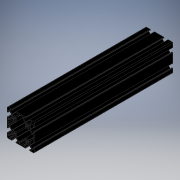
# Autodesk Inventor part: 20-4040-Black-203.2-CL
Saved by Autodesk Inventor 2019 (Build 230136000, 136)
## iProperties
Created: 2022-06-30
Part Number: 20-4040-Black-203.2-CL
Material: Generic
Catalog Web Link: www.cadenas.de
Description: 20-4040, 20-4040-Black-T-Slotted Profile - 20 Series
Vendor: 8020
Document SubType Name: Modeling
Designer: psAdmin
Manufacturer: 8020
Mass: 85.9678 g
Surface Area: 1092.07 cm^2
Volume: 85.9678 cm^3
Density: 1 g/cm^3
Appearance: PSOLRGB-0-0-0
Category: PARTsolutions
Company: 8020
Title: 20-4040-Black-203.2
Author: Cadenas PARTsolutions
Comments: T-Slotted Profile - 20 Series
PSOL_IDENT_0: {$CADENAS_DATA/23d-libs/8020/metric/profiles/20_series/20_4040.prj},206 {VTYP=3D},{NB=20-4040-Black-
PSOL_IDENT_1: 203.2-CL},{LINA=20-4040-Black-203.2},{NN=20-4040, 20-4040-Black},{DATE=31.07.2020 09:21:32},{GEOMDAT
PSOL_IDENT_2: E=09.02.2018 15:36:41},{VERSION=},{LINEID=10},{WBVAR=FIN,LS,L},{WBNUMERIC=L}  {NB=20-4040-Black-203.
PSOL_IDENT_3: 2-CL},{LINA=20-4040-Black-203.2},{KT=DUMMY},{PN=20-4040-Black-203.2},{PN1=20-4040},{FIN=BA},{LS=-CL}
PSOL_IDENT_4: ,{L=203.20},{SERIES=20-4040},{MAT=6105-T5 Aluminum},{W=1.1727},{LALG=[25:6000/0.05]},{MIX=7.8220},{M
PSOL_IDENT_5: IY=7.8220},{EA=4.2221},{COLOR=0,0,0}
NB: 20-4040-Black-203.2-CL
NN: 20-4040, 20-4040-Black
NT: T-Slotted Profile - 20 Series
NBSYN: $PN.$LS.
LINA: 20-4040-Black-203.2
CATALOG: 80/20
PN: 20-4040-Black-203.2
FIN: Black Anodize
LS: Custom Length
L: 203.2
SERIES: 20-4040
MAT: 6105-T5 Aluminum
W: 1.1727
MIX: 7.8220
MIY: 7.8220
EA: 4.2221
SUPPLIER: 8020
ARTICLENO: 20-4040-Black-203.2-CL
BOMINFO: 20-4040-Black-203.2
CREATOR: CADENAS GmbH
Autodesk Inventor part; units mm, degrees
ref_plane "YZ Plane" through (0, 0, 0) normal (1, 0, 0) x (0, 1, 0)
ref_plane "XZ Plane" through (0, 0, 0) normal (0, 1, 0) x (-1, 0, 0)
ref_plane "XY Plane" through (0, 0, 0) normal (0, 0, 1) x (1, 0, 0)
sketch "Sketch_1" plane through (0, 0, 0) normal (0, 0, 1) x (1, 0, 0)
  line L0 (-20, 28.5) -> (-20, 23.138)
  arc A0 (-20, 23.138) -> (-19.492, 22.63) centre (-19.492, 23.138) ccw
  line L1 (-19.492, 22.63) -> (-19.008, 22.63)
  arc A1 (-19.008, 22.63) -> (-18.5, 23.138) centre (-19.008, 23.138) ccw
  line L2 (-18.5, 23.138) -> (-18.5, 25.487)
  arc A2 (-17.992, 25.995) -> (-18.5, 25.487) centre (-17.992, 25.487) ccw
  line L3 (-17.992, 25.995) -> (-17.2659, 25.995)
  arc A3 (-16.9067, 25.8462) -> (-17.2659, 25.995) centre (-17.2659, 25.487) ccw
  line L4 (-16.9067, 25.8462) -> (-13.8038, 22.7433)
  arc A4 (-13.655, 22.3841) -> (-13.8038, 22.7433) centre (-14.163, 22.3841) ccw
  line L5 (-13.655, 22.3841) -> (-13.655, 17.6162)
  arc A5 (-13.8038, 17.257) -> (-13.655, 17.6162) centre (-14.163, 17.6162) ccw
  line L6 (-13.8038, 17.257) -> (-16.907, 14.1538)
  arc A6 (-17.2662, 14.005) -> (-16.907, 14.1538) centre (-17.2662, 14.513) ccw
  line L7 (-17.2662, 14.005) -> (-17.992, 14.005)
  arc A7 (-18.5, 14.513) -> (-17.992, 14.005) centre (-17.992, 14.513) ccw
  line L8 (-18.5, 14.513) -> (-18.5, 16.862)
  arc A8 (-18.5, 16.862) -> (-19.008, 17.37) centre (-19.008, 16.862) ccw
  line L9 (-19.008, 17.37) -> (-19.492, 17.37)
  arc A9 (-19.492, 17.37) -> (-20, 16.862) centre (-19.492, 16.862) ccw
  line L10 (-20, 16.862) -> (-20, 3.138)
  arc A10 (-20, 3.138) -> (-19.492, 2.63) centre (-19.492, 3.138) ccw
  line L11 (-19.492, 2.63) -> (-19.008, 2.63)
  arc A11 (-19.008, 2.63) -> (-18.5, 3.138) centre (-19.008, 3.138) ccw
  line L12 (-18.5, 3.138) -> (-18.5, 5.487)
  arc A12 (-17.992, 5.995) -> (-18.5, 5.487) centre (-17.992, 5.487) ccw
  line L13 (-17.992, 5.995) -> (-17.2662, 5.995)
  arc A13 (-16.907, 5.8462) -> (-17.2662, 5.995) centre (-17.2662, 5.487) ccw
  line L14 (-16.907, 5.8462) -> (-13.8038, 2.743)
  arc A14 (-13.655, 2.3838) -> (-13.8038, 2.743) centre (-14.163, 2.3838) ccw
  line L15 (-13.655, 2.3838) -> (-13.655, -2.3841)
  arc A15 (-13.8038, -2.7433) -> (-13.655, -2.3841) centre (-14.163, -2.3841) ccw
  line L16 (-13.8038, -2.7433) -> (-16.9067, -5.8462)
  arc A16 (-17.2659, -5.995) -> (-16.9067, -5.8462) centre (-17.2659, -5.487) ccw
  line L17 (-17.2659, -5.995) -> (-17.992, -5.995)
  arc A17 (-18.5, -5.487) -> (-17.992, -5.995) centre (-17.992, -5.487) ccw
  line L18 (-18.5, -5.487) -> (-18.5, -3.138)
  arc A18 (-18.5, -3.138) -> (-19.008, -2.63) centre (-19.008, -3.138) ccw
  line L19 (-19.008, -2.63) -> (-19.492, -2.63)
  arc A19 (-19.492, -2.63) -> (-20, -3.138) centre (-19.492, -3.138) ccw
  line L20 (-20, -3.138) -> (-20, -8.5)
  arc A20 (-20, -8.5) -> (-18.5, -10) centre (-18.5, -8.5) ccw
  line L21 (-18.5, -10) -> (-13.138, -10)
  arc A21 (-13.138, -10) -> (-12.63, -9.492) centre (-13.138, -9.492) ccw
  line L22 (-12.63, -9.492) -> (-12.63, -9.008)
  arc A22 (-12.63, -9.008) -> (-13.138, -8.5) centre (-13.138, -9.008) ccw
  line L23 (-13.138, -8.5) -> (-15.487, -8.5)
  arc A23 (-15.995, -7.992) -> (-15.487, -8.5) centre (-15.487, -7.992) ccw
  line L24 (-15.995, -7.992) -> (-15.995, -7.2662)
  arc A24 (-15.8462, -6.907) -> (-15.995, -7.2662) centre (-15.487, -7.2662) ccw
  line L25 (-15.8462, -6.907) -> (-12.743, -3.8038)
  arc A25 (-12.3838, -3.655) -> (-12.743, -3.8038) centre (-12.3838, -4.163) ccw
  line L26 (-12.3838, -3.655) -> (-7.6159, -3.655)
  arc A26 (-7.2567, -3.8038) -> (-7.6159, -3.655) centre (-7.6159, -4.163) ccw
  line L27 (-7.2567, -3.8038) -> (-4.1538, -6.9067)
  arc A27 (-4.005, -7.2659) -> (-4.1538, -6.9067) centre (-4.513, -7.2659) ccw
  line L28 (-4.005, -7.2659) -> (-4.005, -7.992)
  arc A28 (-4.513, -8.5) -> (-4.005, -7.992) centre (-4.513, -7.992) ccw
  line L29 (-4.513, -8.5) -> (-6.862, -8.5)
  arc A29 (-6.862, -8.5) -> (-7.37, -9.008) centre (-6.862, -9.008) ccw
  line L30 (-7.37, -9.008) -> (-7.37, -9.492)
  arc A30 (-7.37, -9.492) -> (-6.862, -10) centre (-6.862, -9.492) ccw
  line L31 (-6.862, -10) -> (6.862, -10)
  arc A31 (6.862, -10) -> (7.37, -9.492) centre (6.862, -9.492) ccw
  line L32 (7.37, -9.492) -> (7.37, -9.008)
  arc A32 (7.37, -9.008) -> (6.862, -8.5) centre (6.862, -9.008) ccw
  line L33 (6.862, -8.5) -> (4.513, -8.5)
  arc A33 (4.005, -7.992) -> (4.513, -8.5) centre (4.513, -7.992) ccw
  line L34 (4.005, -7.992) -> (4.005, -7.2659)
  arc A34 (4.1538, -6.9067) -> (4.005, -7.2659) centre (4.513, -7.2659) ccw
  line L35 (4.1538, -6.9067) -> (7.2567, -3.8038)
  arc A35 (7.6159, -3.655) -> (7.2567, -3.8038) centre (7.6159, -4.163) ccw
  line L36 (7.6159, -3.655) -> (12.3838, -3.655)
  arc A36 (12.743, -3.8038) -> (12.3838, -3.655) centre (12.3838, -4.163) ccw
  line L37 (12.743, -3.8038) -> (15.8462, -6.907)
  arc A37 (15.995, -7.2662) -> (15.8462, -6.907) centre (15.487, -7.2662) ccw
  line L38 (15.995, -7.2662) -> (15.995, -7.992)
  arc A38 (15.487, -8.5) -> (15.995, -7.992) centre (15.487, -7.992) ccw
  line L39 (15.487, -8.5) -> (13.138, -8.5)
  arc A39 (13.138, -8.5) -> (12.63, -9.008) centre (13.138, -9.008) ccw
  line L40 (12.63, -9.008) -> (12.63, -9.492)
  arc A40 (12.63, -9.492) -> (13.138, -10) centre (13.138, -9.492) ccw
  line L41 (13.138, -10) -> (18.5, -10)
  arc A41 (18.5, -10) -> (20, -8.5) centre (18.5, -8.5) ccw
  line L42 (20, -8.5) -> (20, -3.138)
  arc A42 (20, -3.138) -> (19.492, -2.63) centre (19.492, -3.138) ccw
  line L43 (19.492, -2.63) -> (19.008, -2.63)
  arc A43 (19.008, -2.63) -> (18.5, -3.138) centre (19.008, -3.138) ccw
  line L44 (18.5, -3.138) -> (18.5, -5.487)
  arc A44 (17.992, -5.995) -> (18.5, -5.487) centre (17.992, -5.487) ccw
  line L45 (17.992, -5.995) -> (17.2659, -5.995)
  arc A45 (16.9067, -5.8462) -> (17.2659, -5.995) centre (17.2659, -5.487) ccw
  line L46 (16.9067, -5.8462) -> (13.8038, -2.7433)
  arc A46 (13.655, -2.3841) -> (13.8038, -2.7433) centre (14.163, -2.3841) ccw
  line L47 (13.655, -2.3841) -> (13.655, 2.3838)
  arc A47 (13.8038, 2.743) -> (13.655, 2.3838) centre (14.163, 2.3838) ccw
  line L48 (13.8038, 2.743) -> (16.907, 5.8462)
  arc A48 (17.2662, 5.995) -> (16.907, 5.8462) centre (17.2662, 5.487) ccw
  line L49 (17.2662, 5.995) -> (17.992, 5.995)
  arc A49 (18.5, 5.487) -> (17.992, 5.995) centre (17.992, 5.487) ccw
  line L50 (18.5, 5.487) -> (18.5, 3.138)
  arc A50 (18.5, 3.138) -> (19.008, 2.63) centre (19.008, 3.138) ccw
  line L51 (19.008, 2.63) -> (19.492, 2.63)
  arc A51 (19.492, 2.63) -> (20, 3.138) centre (19.492, 3.138) ccw
  line L52 (20, 3.138) -> (20, 16.862)
  arc A52 (20, 16.862) -> (19.492, 17.37) centre (19.492, 16.862) ccw
  line L53 (19.492, 17.37) -> (19.008, 17.37)
  arc A53 (19.008, 17.37) -> (18.5, 16.862) centre (19.008, 16.862) ccw
  line L54 (18.5, 16.862) -> (18.5, 14.513)
  arc A54 (17.992, 14.005) -> (18.5, 14.513) centre (17.992, 14.513) ccw
  line L55 (17.992, 14.005) -> (17.2662, 14.005)
  arc A55 (16.907, 14.1538) -> (17.2662, 14.005) centre (17.2662, 14.513) ccw
  line L56 (16.907, 14.1538) -> (13.8038, 17.257)
  arc A56 (13.655, 17.6162) -> (13.8038, 17.257) centre (14.163, 17.6162) ccw
  line L57 (13.655, 17.6162) -> (13.655, 22.3841)
  arc A57 (13.8038, 22.7433) -> (13.655, 22.3841) centre (14.163, 22.3841) ccw
  line L58 (13.8038, 22.7433) -> (16.9067, 25.8462)
  arc A58 (17.2659, 25.995) -> (16.9067, 25.8462) centre (17.2659, 25.487) ccw
  line L59 (17.2659, 25.995) -> (17.992, 25.995)
  arc A59 (18.5, 25.487) -> (17.992, 25.995) centre (17.992, 25.487) ccw
  line L60 (18.5, 25.487) -> (18.5, 23.138)
  arc A60 (18.5, 23.138) -> (19.008, 22.63) centre (19.008, 23.138) ccw
  line L61 (19.008, 22.63) -> (19.492, 22.63)
  arc A61 (19.492, 22.63) -> (20, 23.138) centre (19.492, 23.138) ccw
  line L62 (20, 23.138) -> (20, 28.5)
  arc A62 (20, 28.5) -> (18.5, 30) centre (18.5, 28.5) ccw
  line L63 (18.5, 30) -> (13.138, 30)
  arc A63 (13.138, 30) -> (12.63, 29.492) centre (13.138, 29.492) ccw
  line L64 (12.63, 29.492) -> (12.63, 29.008)
  arc A64 (12.63, 29.008) -> (13.138, 28.5) centre (13.138, 29.008) ccw
  line L65 (13.138, 28.5) -> (15.487, 28.5)
  arc A65 (15.995, 27.992) -> (15.487, 28.5) centre (15.487, 27.992) ccw
  line L66 (15.995, 27.992) -> (15.995, 27.2662)
  arc A66 (15.8462, 26.907) -> (15.995, 27.2662) centre (15.487, 27.2662) ccw
  line L67 (15.8462, 26.907) -> (12.743, 23.8038)
  arc A67 (12.3838, 23.655) -> (12.743, 23.8038) centre (12.3838, 24.163) ccw
  line L68 (12.3838, 23.655) -> (7.6159, 23.655)
  arc A68 (7.2567, 23.8038) -> (7.6159, 23.655) centre (7.6159, 24.163) ccw
  line L69 (7.2567, 23.8038) -> (4.1538, 26.9067)
  arc A69 (4.005, 27.2659) -> (4.1538, 26.9067) centre (4.513, 27.2659) ccw
  line L70 (4.005, 27.2659) -> (4.005, 27.992)
  arc A70 (4.513, 28.5) -> (4.005, 27.992) centre (4.513, 27.992) ccw
  line L71 (4.513, 28.5) -> (6.862, 28.5)
  arc A71 (6.862, 28.5) -> (7.37, 29.008) centre (6.862, 29.008) ccw
  line L72 (7.37, 29.008) -> (7.37, 29.492)
  arc A72 (7.37, 29.492) -> (6.862, 30) centre (6.862, 29.492) ccw
  line L73 (6.862, 30) -> (-6.862, 30)
  arc A73 (-6.862, 30) -> (-7.37, 29.492) centre (-6.862, 29.492) ccw
  line L74 (-7.37, 29.492) -> (-7.37, 29.008)
  arc A74 (-7.37, 29.008) -> (-6.862, 28.5) centre (-6.862, 29.008) ccw
  line L75 (-6.862, 28.5) -> (-4.513, 28.5)
  arc A75 (-4.005, 27.992) -> (-4.513, 28.5) centre (-4.513, 27.992) ccw
  line L76 (-4.005, 27.992) -> (-4.005, 27.2659)
  arc A76 (-4.1538, 26.9067) -> (-4.005, 27.2659) centre (-4.513, 27.2659) ccw
  line L77 (-4.1538, 26.9067) -> (-7.2567, 23.8038)
  arc A77 (-7.6159, 23.655) -> (-7.2567, 23.8038) centre (-7.6159, 24.163) ccw
  line L78 (-7.6159, 23.655) -> (-12.3838, 23.655)
  arc A78 (-12.743, 23.8038) -> (-12.3838, 23.655) centre (-12.3838, 24.163) ccw
  line L79 (-12.743, 23.8038) -> (-15.8462, 26.907)
  arc A79 (-15.995, 27.2662) -> (-15.8462, 26.907) centre (-15.487, 27.2662) ccw
  line L80 (-15.995, 27.2662) -> (-15.995, 27.992)
  arc A80 (-15.487, 28.5) -> (-15.995, 27.992) centre (-15.487, 27.992) ccw
  line L81 (-15.487, 28.5) -> (-13.138, 28.5)
  arc A81 (-13.138, 28.5) -> (-12.63, 29.008) centre (-13.138, 29.008) ccw
  line L82 (-12.63, 29.008) -> (-12.63, 29.492)
  arc A82 (-12.63, 29.492) -> (-13.138, 30) centre (-13.138, 29.492) ccw
  line L83 (-13.138, 30) -> (-18.5, 30)
  arc A83 (-18.5, 30) -> (-20, 28.5) centre (-18.5, 28.5) ccw
  arc A84 (8.0642, -0.8037) -> (7.6955, -2.1245) centre (8.252, -1.568) ccw
  line L84 (7.6955, -2.1245) -> (7.8755, -2.3045)
  arc A85 (7.8755, -2.3045) -> (9.1963, -1.9358) centre (8.432, -1.748) ccw
  arc A86 (9.1963, -1.9358) -> (10.8037, -1.9358) centre (10, 0) ccw
  arc A87 (10.8037, -1.9358) -> (12.1245, -2.3045) centre (11.568, -1.748) ccw
  line L85 (12.1245, -2.3045) -> (12.3045, -2.1245)
  arc A88 (12.3045, -2.1245) -> (11.9358, -0.8037) centre (11.748, -1.568) ccw
  arc A89 (11.9358, -0.8037) -> (11.9358, 0.8037) centre (10, 0) ccw
  arc A90 (11.9358, 0.8037) -> (12.3045, 2.1245) centre (11.748, 1.568) ccw
  line L86 (12.3045, 2.1245) -> (12.1245, 2.3045)
  arc A91 (12.1245, 2.3045) -> (10.8037, 1.9358) centre (11.568, 1.748) ccw
  arc A92 (10.8037, 1.9358) -> (9.1963, 1.9358) centre (10, 0) ccw
  arc A93 (9.1963, 1.9358) -> (7.8755, 2.3045) centre (8.432, 1.748) ccw
  line L87 (7.8755, 2.3045) -> (7.6955, 2.1245)
  arc A94 (7.6955, 2.1245) -> (8.0642, 0.8037) centre (8.252, 1.568) ccw
  arc A95 (8.0642, 0.8037) -> (8.0642, -0.8037) centre (10, 0) ccw
  arc A96 (7.6955, 22.1245) -> (8.0642, 20.8037) centre (8.252, 21.568) ccw
  arc A97 (8.0642, 20.8037) -> (8.0642, 19.1963) centre (10, 20) ccw
  arc A98 (8.0642, 19.1963) -> (7.6955, 17.8755) centre (8.252, 18.432) ccw
  line L88 (7.6955, 17.8755) -> (7.8755, 17.6955)
  arc A99 (7.8755, 17.6955) -> (9.1963, 18.0642) centre (8.432, 18.252) ccw
  arc A100 (9.1963, 18.0642) -> (10.8037, 18.0642) centre (10, 20) ccw
  arc A101 (10.8037, 18.0642) -> (12.1245, 17.6955) centre (11.568, 18.252) ccw
  line L89 (12.1245, 17.6955) -> (12.3045, 17.8755)
  arc A102 (12.3045, 17.8755) -> (11.9358, 19.1963) centre (11.748, 18.432) ccw
  arc A103 (11.9358, 19.1963) -> (11.9358, 20.8037) centre (10, 20) ccw
  arc A104 (11.9358, 20.8037) -> (12.3045, 22.1245) centre (11.748, 21.568) ccw
  line L90 (12.3045, 22.1245) -> (12.1245, 22.3045)
  arc A105 (12.1245, 22.3045) -> (10.8037, 21.9358) centre (11.568, 21.748) ccw
  arc A106 (10.8037, 21.9358) -> (9.1963, 21.9358) centre (10, 20) ccw
  arc A107 (9.1963, 21.9358) -> (7.8755, 22.3045) centre (8.432, 21.748) ccw
  line L91 (7.8755, 22.3045) -> (7.6955, 22.1245)
  arc A108 (-11.9358, -0.8037) -> (-12.3045, -2.1245) centre (-11.748, -1.568) ccw
  line L92 (-12.3045, -2.1245) -> (-12.1245, -2.3045)
  arc A109 (-12.1245, -2.3045) -> (-10.8037, -1.9358) centre (-11.568, -1.748) ccw
  arc A110 (-10.8037, -1.9358) -> (-9.1963, -1.9358) centre (-10, 0) ccw
  arc A111 (-9.1963, -1.9358) -> (-7.8755, -2.3045) centre (-8.432, -1.748) ccw
  line L93 (-7.8755, -2.3045) -> (-7.6955, -2.1245)
  arc A112 (-7.6955, -2.1245) -> (-8.0642, -0.8037) centre (-8.252, -1.568) ccw
  arc A113 (-8.0642, -0.8037) -> (-8.0642, 0.8037) centre (-10, 0) ccw
  arc A114 (-8.0642, 0.8037) -> (-7.6955, 2.1245) centre (-8.252, 1.568) ccw
  line L94 (-7.6955, 2.1245) -> (-7.8755, 2.3045)
  arc A115 (-7.8755, 2.3045) -> (-9.1963, 1.9358) centre (-8.432, 1.748) ccw
  arc A116 (-9.1963, 1.9358) -> (-10.8037, 1.9358) centre (-10, 0) ccw
  arc A117 (-10.8037, 1.9358) -> (-12.1245, 2.3045) centre (-11.568, 1.748) ccw
  line L95 (-12.1245, 2.3045) -> (-12.3045, 2.1245)
  arc A118 (-12.3045, 2.1245) -> (-11.9358, 0.8037) centre (-11.748, 1.568) ccw
  arc A119 (-11.9358, 0.8037) -> (-11.9358, -0.8037) centre (-10, 0) ccw
  arc A120 (-12.3045, 22.1245) -> (-11.9358, 20.8037) centre (-11.748, 21.568) ccw
  arc A121 (-11.9358, 20.8037) -> (-11.9358, 19.1963) centre (-10, 20) ccw
  arc A122 (-11.9358, 19.1963) -> (-12.3045, 17.8755) centre (-11.748, 18.432) ccw
  line L96 (-12.3045, 17.8755) -> (-12.1245, 17.6955)
  arc A123 (-12.1245, 17.6955) -> (-10.8037, 18.0642) centre (-11.568, 18.252) ccw
  arc A124 (-10.8037, 18.0642) -> (-9.1963, 18.0642) centre (-10, 20) ccw
  arc A125 (-9.1963, 18.0642) -> (-7.8755, 17.6955) centre (-8.432, 18.252) ccw
  line L97 (-7.8755, 17.6955) -> (-7.6955, 17.8755)
  arc A126 (-7.6955, 17.8755) -> (-8.0642, 19.1963) centre (-8.252, 18.432) ccw
  arc A127 (-8.0642, 19.1963) -> (-8.0642, 20.8037) centre (-10, 20) ccw
  arc A128 (-8.0642, 20.8037) -> (-7.6955, 22.1245) centre (-8.252, 21.568) ccw
  line L98 (-7.6955, 22.1245) -> (-7.8755, 22.3045)
  arc A129 (-7.8755, 22.3045) -> (-9.1963, 21.9358) centre (-8.432, 21.748) ccw
  arc A130 (-9.1963, 21.9358) -> (-10.8037, 21.9358) centre (-10, 20) ccw
  arc A131 (-10.8037, 21.9358) -> (-12.1245, 22.3045) centre (-11.568, 21.748) ccw
  line L99 (-12.1245, 22.3045) -> (-12.3045, 22.1245)
  arc A132 (-18.5, 8.003) -> (-17.992, 7.495) centre (-17.992, 8.003) ccw
  line L100 (-17.992, 7.495) -> (-16.6449, 7.495)
  arc A133 (-16.2857, 7.3462) -> (-16.6449, 7.495) centre (-16.6449, 6.987) ccw
  line L101 (-16.2857, 7.3462) -> (-12.7433, 3.8038)
  arc A134 (-12.7433, 3.8038) -> (-12.3841, 3.655) centre (-12.3841, 4.163) ccw
  line L102 (-12.3841, 3.655) -> (-7.488, 3.655)
  arc A135 (-6.345, 2.512) -> (-7.488, 3.655) centre (-7.488, 2.512) ccw
  line L103 (-6.345, 2.512) -> (-6.345, -2.3838)
  arc A136 (-6.345, -2.3838) -> (-6.1962, -2.743) centre (-5.837, -2.3838) ccw
  line L104 (-6.1962, -2.743) -> (-2.6538, -6.2854)
  arc A137 (-2.505, -6.6446) -> (-2.6538, -6.2854) centre (-3.013, -6.6446) ccw
  line L105 (-2.505, -6.6446) -> (-2.505, -7.992)
  arc A138 (-2.505, -7.992) -> (-1.997, -8.5) centre (-1.997, -7.992) ccw
  line L106 (-1.997, -8.5) -> (1.997, -8.5)
  arc A139 (1.997, -8.5) -> (2.505, -7.992) centre (1.997, -7.992) ccw
  line L107 (2.505, -7.992) -> (2.505, -6.6446)
  arc A140 (2.6538, -6.2854) -> (2.505, -6.6446) centre (3.013, -6.6446) ccw
  line L108 (2.6538, -6.2854) -> (6.1962, -2.743)
  arc A141 (6.1962, -2.743) -> (6.345, -2.3838) centre (5.837, -2.3838) ccw
  line L109 (6.345, -2.3838) -> (6.345, 2.512)
  arc A142 (7.488, 3.655) -> (6.345, 2.512) centre (7.488, 2.512) ccw
  line L110 (7.488, 3.655) -> (12.3841, 3.655)
  arc A143 (12.3841, 3.655) -> (12.7433, 3.8038) centre (12.3841, 4.163) ccw
  line L111 (12.7433, 3.8038) -> (16.2857, 7.3462)
  arc A144 (16.6449, 7.495) -> (16.2857, 7.3462) centre (16.6449, 6.987) ccw
  line L112 (16.6449, 7.495) -> (17.992, 7.495)
  arc A145 (17.992, 7.495) -> (18.5, 8.003) centre (17.992, 8.003) ccw
  line L113 (18.5, 8.003) -> (18.5, 11.997)
  arc A146 (18.5, 11.997) -> (17.992, 12.505) centre (17.992, 11.997) ccw
  line L114 (17.992, 12.505) -> (16.6449, 12.505)
  arc A147 (16.2857, 12.6538) -> (16.6449, 12.505) centre (16.6449, 13.013) ccw
  line L115 (16.2857, 12.6538) -> (12.7433, 16.1962)
  arc A148 (12.7433, 16.1962) -> (12.3841, 16.345) centre (12.3841, 15.837) ccw
  line L116 (12.3841, 16.345) -> (7.488, 16.345)
  arc A149 (6.345, 17.488) -> (7.488, 16.345) centre (7.488, 17.488) ccw
  line L117 (6.345, 17.488) -> (6.345, 22.3838)
  arc A150 (6.345, 22.3838) -> (6.1962, 22.743) centre (5.837, 22.3838) ccw
  line L118 (6.1962, 22.743) -> (2.6538, 26.2854)
  arc A151 (2.505, 26.6446) -> (2.6538, 26.2854) centre (3.013, 26.6446) ccw
  line L119 (2.505, 26.6446) -> (2.505, 27.992)
  arc A152 (2.505, 27.992) -> (1.997, 28.5) centre (1.997, 27.992) ccw
  line L120 (1.997, 28.5) -> (-1.997, 28.5)
  arc A153 (-1.997, 28.5) -> (-2.505, 27.992) centre (-1.997, 27.992) ccw
  line L121 (-2.505, 27.992) -> (-2.505, 26.6446)
  arc A154 (-2.6538, 26.2854) -> (-2.505, 26.6446) centre (-3.013, 26.6446) ccw
  line L122 (-2.6538, 26.2854) -> (-6.1962, 22.743)
  arc A155 (-6.1962, 22.743) -> (-6.345, 22.3838) centre (-5.837, 22.3838) ccw
  line L123 (-6.345, 22.3838) -> (-6.345, 17.488)
  arc A156 (-7.488, 16.345) -> (-6.345, 17.488) centre (-7.488, 17.488) ccw
  line L124 (-7.488, 16.345) -> (-12.3841, 16.345)
  arc A157 (-12.3841, 16.345) -> (-12.7433, 16.1962) centre (-12.3841, 15.837) ccw
  line L125 (-12.7433, 16.1962) -> (-16.2857, 12.6538)
  arc A158 (-16.6449, 12.505) -> (-16.2857, 12.6538) centre (-16.6449, 13.013) ccw
  line L126 (-16.6449, 12.505) -> (-17.992, 12.505)
  arc A159 (-17.992, 12.505) -> (-18.5, 11.997) centre (-17.992, 11.997) ccw
  line L127 (-18.5, 11.997) -> (-18.5, 8.003)
  constraints: 320 point on circle, 256 end point, 160 centre point
extrude "Extrusion1" add sketch "Sketch_1" against normal blind 203.2
body "Solid1"
